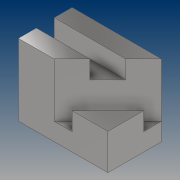
# Autodesk Inventor part: 17
Saved by Autodesk Inventor 2020.2 (Build 242310000, 310)
## iProperties
Created: 2020-09-17
Part Number: 17
Material: 鋼、碳鋼
Document SubType Name: Modeling
Designer: user
Density: 7.85 g/cm^3
Appearance: 半拋光
Mass: 353.25 g
Surface Area: 100.142 cm^2
Volume: 45 cm^3
Author: user
Autodesk Inventor part; units mm, degrees
ref_plane "YZ Plane" through (0, 0, 0) normal (1, 0, 0) x (0, 1, 0)
ref_plane "XZ Plane" through (0, 0, 0) normal (0, 1, 0) x (-1, 0, 0)
ref_plane "XY Plane" through (0, 0, 0) normal (0, 0, 1) x (1, 0, 0)
sketch "草圖1" plane through (0, 0, 0) normal (0, 1, 0) x (-1, 0, 0)
  line L0 (0, 0) -> (-50, 0)
  line L1 (-50, 0) -> (-50, -30)
  line L2 (-50, -30) -> (0, -30)
  line L3 (0, -30) -> (0, 0)
  dimension "d0" = 50
  dimension "d1" = 30
  constraints: 8 end point, 2 parallel, 1 horizontal, 1 perpendicular
  measures "d0" distance of L0.start L0.end
  measures "d1" distance of L2.end L0.start
extrude "擠出1" add sketch "草圖1" along normal blind 40
sketch "草圖2" plane through (0, 0, -30) normal (-1, 0, 0) x (0, 0, 1)
  line L0 (0, 0) -> (0, 40) projected
  line L1 (0, 40) -> (30, 40) projected
  line L2 (30, 40) -> (30, 0) projected
  line L3 (30, 0) -> (0, 0) projected
  line L4 (10, 40) -> (20, 40)
  line L5 (20, 40) -> (20, 30)
  line L6 (20, 30) -> (10, 30)
  line L7 (10, 30) -> (10, 40)
  point P0 (15, 40)
  dimension "d4" = 10
  dimension "d5" = 10
  constraints: 8 end point, 2 midpoint, 2 parallel, 1 horizontal, 1 perpendicular
  measures "d4" distance of L5.end L6.end
  measures "d5" distance of L4.end L5.end
extrude "擠出2" cut sketch "草圖2" against normal blind 70.25 contours L1 L5 L6 L7
sketch "草圖3" plane through (0, 40, 0) normal (0, 1, 0) x (1, 0, 0)
  line L0 (0, 10) -> (50, 10) projected
  line L1 (50, 10) -> (50, 0) projected
  line L2 (50, 0) -> (0, 0) projected
  line L3 (0, 0) -> (0, 10) projected
  line L4 (50, 20) -> (0, 20) projected
  line L5 (0, 20) -> (0, 30) projected
  line L6 (0, 30) -> (50, 30) projected
  line L7 (50, 30) -> (50, 20) projected
  line L8 (50, 0) -> (50, 30) projected
  line L9 (50, 30) -> (20, 0)
  line L10 (30, 0) -> (50, 20)
  line L11 (0, 20) -> (50, 20) projected
  dimension "d8" = 30
  dimension "d10" = 20
  constraints: 4 end point, 3 point on line, 1 parallel
  measures "d8" distance from line of L1 L9.end
  measures "d10" distance from line of L1 L10.start
extrude "擠出3" cut sketch "草圖3" against normal blind 30 contours L9 L4 L10 L0 | L0 L10 L2 L9 | L9 L7 L4
sketch "草圖4" plane through (0, 40, 0) normal (0, 1, 0) x (1, 0, 0)
  line L0 (50, 30) -> (40, 20) projected
  line L1 (40, 20) -> (0, 20) projected
  line L2 (0, 20) -> (0, 30) projected
  line L3 (0, 30) -> (50, 30) projected
  line L4 (30, 10) -> (20, 0) projected
  line L5 (20, 0) -> (0, 0) projected
  line L6 (0, 0) -> (0, 10) projected
  line L7 (0, 10) -> (30, 10) projected
  line L8 (50, 10) -> (50, 0) projected
  line L9 (50, 0) -> (30, 0) projected
  line L10 (30, 0) -> (40, 10) projected
  line L11 (40, 10) -> (50, 10) projected
  line L12 (50, 20) -> (40, 10) projected
  line L13 (40, 10) -> (50, 10) projected
  line L14 (50, 20) -> (50, 10) projected
extrude "擠出4" cut sketch "草圖4" against normal blind 20 contours L8 L9 L10 L11 | L11 L12 L14
